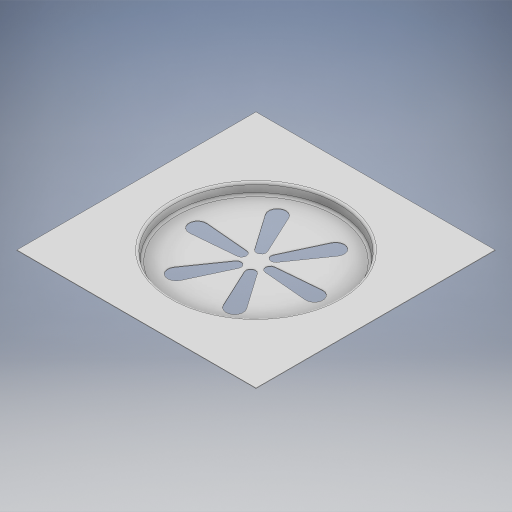
# Autodesk Inventor part: A2.2-big-punch-3
Saved by Autodesk Inventor 2024 (Build 280153000, 153)
## iProperties
Created: 2024-02-18
Part Number: A2.2-big-punch-3
Material: Generic
Document SubType Name: Sheet Metal
Designer: Alex
Density: 1 g/cm^3
Sheet Metal Rule: Default_mm
Appearance: Default
Author: Alex
Autodesk Inventor part; units mm, degrees
ref_plane "YZ Plane" through (0, 0, 0) normal (1, 0, 0) x (0, 1, 0)
ref_plane "XZ Plane" through (0, 0, 0) normal (0, 1, 0) x (-1, 0, 0)
sketch "Sketch1" plane through (0, 0, 0) normal (0, 1, 0) x (-1, 0, 0)
  line L0 (0, 0) -> (250, 0)
  line L1 (250, 0) -> (250, -250)
  line L2 (250, -250) -> (0, -250)
  line L3 (0, -250) -> (0, 0)
  dimension "d0" = 250
  dimension "d1" = 250
  measures "d0" distance of L1.end L2.end
  measures "d1" distance of L0.end L1.end
extrude "Plate1" add sketch "Sketch1" along normal blind 0.5
sketch "Sketch2" plane through (0, 0.5, 0) normal (0, 1, 0) x (1, 0, 0)
  line L0 (0, 0) -> (-250, 0) construction
  line L1 (0, 250) -> (0, 0) construction
  circle A0 centre (-125, 125) radius 90
  line L2 (-125, 125) -> (-215, 125) construction
  line L3 (-125, 125) -> (-125, 35) construction
  circle A1 centre (-125, 125) radius 87
  dimension "d3" = 125
  dimension "d4" = 125
  dimension "d5" = 180
  dimension "d29" = 3
  constraints: 4 end point, 2 centre point, 2 point on circle, 1 coincident, 1 horizontal, 1 vertical
  measures "d3" distance from line of L1 point (-125, 125)
  measures "d4" distance from line of point (-125, 125) L0
  measures "d5" diameter of A0
  measures "d29" radial gap between concentric circles of A0 A1
sketch "Sketch2 outline for Extrusion5" plane through (0, 0.5, 0) normal (0, 1, 0) x (1, 0, 0)
  circle A0 centre (-125, 125) radius 90
extrude "Extrusion5" add sketch "Sketch2 outline for Extrusion5" against normal blind 11 draft -10
extrude "Extrusion6" cut sketch "Sketch2" against normal blind 10.5 draft -10 contours A1
fillet "Fillet1" radius 2.5 4 edges at (-212, 0.5, -125) (-214.9118, 0, -125) (-213.0604, -10.5, -125) (-210.1486, -10, -125)
ref_plane "Work Plane6" through (-125, -10, -125) normal (0, 1, 0) x (-1, 0, 0)
ref_plane "Work Plane5" through (-125, 0.5, -125) normal (0, 1, 0) x (-1, 0, 0)
sketch "Sketch6" plane through (-125, -10, -125) normal (0, 1, 0) x (-1, 0, 0)
  line L0 (0, 0) -> (90, 0) construction
  line L1 (0, 0) -> (0, 90) construction
  arc A0 (60.217391, -8.965909) -> (60.217391, 8.965909) centre (61, 0) ccw
  arc A1 (14.565217, 4.981061) -> (14.565217, -4.981061) centre (15, 0) ccw
  line L2 (14.565217, -4.981061) -> (60.217391, -8.965909)
  line L3 (14.565217, 4.981061) -> (60.217391, 8.965909)
  line L4 (10, 0) -> (70, 0) construction
  arc A2 (2.968884, 15.104379) -> (11.596334, 10.123318) centre (7.5, 12.990381) ccw
  line L5 (2.968884, 15.104379) -> (22.343991, 56.632745)
  line L6 (5, 8.660254) -> (35, 60.621778) construction
  line L7 (11.596334, 10.123318) -> (37.873401, 47.666836)
  arc A3 (37.873401, 47.666836) -> (22.343991, 56.632745) centre (30.5, 52.82755) ccw
  arc A4 (-11.596334, 10.123318) -> (-2.968884, 15.104379) centre (-7.5, 12.990381) ccw
  line L8 (-11.596334, 10.123318) -> (-37.873401, 47.666836)
  line L9 (-5, 8.660254) -> (-35, 60.621778) construction
  line L10 (-2.968884, 15.104379) -> (-22.343991, 56.632745)
  arc A5 (-22.343991, 56.632745) -> (-37.873401, 47.666836) centre (-30.5, 52.82755) ccw
  arc A6 (-14.565217, -4.981061) -> (-14.565217, 4.981061) centre (-15, 0) ccw
  line L11 (-14.565217, -4.981061) -> (-60.217391, -8.965909)
  line L12 (-10, 0) -> (-70, 0) construction
  line L13 (-14.565217, 4.981061) -> (-60.217391, 8.965909)
  arc A7 (-60.217391, 8.965909) -> (-60.217391, -8.965909) centre (-61, 0) ccw
  arc A8 (-2.968884, -15.104379) -> (-11.596334, -10.123318) centre (-7.5, -12.990381) ccw
  line L14 (-2.968884, -15.104379) -> (-22.343991, -56.632745)
  line L15 (-5, -8.660254) -> (-35, -60.621778) construction
  line L16 (-11.596334, -10.123318) -> (-37.873401, -47.666836)
  arc A9 (-37.873401, -47.666836) -> (-22.343991, -56.632745) centre (-30.5, -52.82755) ccw
  arc A10 (11.596334, -10.123318) -> (2.968884, -15.104379) centre (7.5, -12.990381) ccw
  line L17 (11.596334, -10.123318) -> (37.873401, -47.666836)
  line L18 (5, -8.660254) -> (35, -60.621778) construction
  line L19 (2.968884, -15.104379) -> (22.343991, -56.632745)
  arc A11 (22.343991, -56.632745) -> (37.873401, -47.666836) centre (30.5, -52.82755) ccw
  point P0 (-125, 125)
  dimension "d38" = 5
  dimension "d39" = 9
  dimension "d40" = 15
  dimension "d41" = 60
  dimension "d42" = 360
  constraints: 36 end point, 26 point on circle, 12 centre point, 6 point on line, 4 tangent, 1 coincident, 1 horizontal, 1 horizontal alignment, 79 other
  measures "d38" radius of A1
  measures "d39" radius of A0
  measures "d40" distance of A1.centre point (0, 0)
  measures "d41" distance of L4.start L4.end
extrude "Extrusion7" cut sketch "Sketch6" against normal blind 0.5
equation "\"d32\" = Profile - Thickness"
equation "\"d34\" = 5 * Thickness"
equation "\"d43\" = Thickness"
equation "\"d2\" = Thickness"
equation "\"BendRadius\" = Thickness"
equation "\"BendReliefWidth\" = Thickness"
equation "\"BendReliefDepth\" = 0.5 * Thickness"
equation "\"CornerReliefSize\" = 4 * Thickness"
equation "\"MinimumRemnant\" = 2 * Thickness"
equation "\"TransitionRadius\" = BendRadius"
equation "\"JacobiRadiusSize\" = BendRadius"
equation "\"GapSize\" = Thickness"
equation "\"Profile\" = 11"
equation "\"Thickness\" = 0.5"
body "Solid1"
